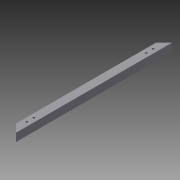
# Autodesk Inventor part: Square Tube 2
Saved by Autodesk Inventor 2013 (Build 170138000, 138)
## iProperties
Created: 2013-01-24
Part Number: Square Tube 2
Material: Generic
Document SubType Name: Modeling
Designer: actoennies
Density: 1 g/cm^3
Mass: 70.1426 g
Surface Area: 893.355 cm^2
Volume: 70.1426 cm^3
Author: actoennies
Autodesk Inventor part; units mm, degrees
ref_plane "YZ Plane" through (0, 0, 0) normal (1, 0, 0) x (0, 1, 0)
ref_plane "XZ Plane" through (0, 0, 0) normal (0, 1, 0) x (-1, 0, 0)
ref_plane "XY Plane" through (0, 0, 0) normal (0, 0, 1) x (1, 0, 0)
sketch "Sketch1" plane through (0, 0, 0) normal (0, 0, 1) x (1, 0, 0)
  line L0 (0, 0) -> (25.4, 0)
  line L1 (25.4, 0) -> (25.4, 25.4)
  line L2 (25.4, 25.4) -> (0, 25.4)
  line L3 (0, 25.4) -> (0, 0)
  line L4 (1.5875, 23.8125) -> (23.8125, 23.8125)
  line L5 (23.8125, 23.8125) -> (23.8125, 1.5875)
  line L6 (23.8125, 1.5875) -> (1.5875, 1.5875)
  line L7 (1.5875, 1.5875) -> (1.5875, 23.8125)
  dimension "d0" = 25.4
  dimension "d2" = 25.4
  dimension "d3" = 1.5875
  constraints: 16 end point, 4 parallel, 2 perpendicular, 1 horizontal, 3 other
  measures "d0" distance of L1.end L2.end
  measures "d2" distance of L0.end L1.end
  measures "d3" distance between parallel lines of L2 L4
extrude "Extrusion1" add sketch "Sketch1" along normal blind 495.3
sketch "Sketch2" plane through (0, 25.4, 0) normal (0, 1, 0) x (1, 0, 0)
  line L0 (25.4, 0) -> (0, 0) projected
  line L1 (0, 0) -> (0, -495.3) projected
  line L2 (25.4, -495.3) -> (0, -495.3) projected
  line L3 (25.4, 0) -> (25.4, -495.3) projected
  line L4 (25.4, -495.3) -> (0, -469.9)
  line L5 (25.4, 0) -> (0, -25.4)
  dimension "d6" = 135
  dimension "d7" = 45
  constraints: 4 end point, 2 point on line
  measures "d6" angle of L3 L5
  measures "d7" angle of L3 L4
extrude "Extrusion2" cut sketch "Sketch2" against normal blind 495.3 contours L5 L1 L0 | L2 L1 L4
sketch "Sketch3" plane through (25.4, 0, 0) normal (0, -1, 0) x (1, 0, 0)
  circle A0 centre (-12.7, 69.85) radius 3.3782 projected
  circle A1 centre (-12.7, 47.625) radius 3.3782 projected
  circle A2 centre (-12.7, 425.45) radius 3.3782 projected
  circle A3 centre (-12.7, 447.675) radius 3.3782 projected
  point P0 (-25.4, 0)
extrude "Extrusion3" cut sketch "Sketch3" against normal blind 25.4
sketch "Sketch4" plane through (0, 0, 25.4) normal (-1, 0, 0) x (0, 0, 1)
  circle A0 centre (431.8, 12.7) radius 3.3782 projected
  circle A1 centre (381, 12.7) radius 3.3782 projected
  circle A2 centre (12.7, 12.7) radius 3.3782 projected
  circle A3 centre (63.5, 12.7) radius 3.3782 projected
  point P0 (-25.4, 0)
extrude "Extrusion4" cut sketch "Sketch4" against normal blind 25.4
body "Solid1"
